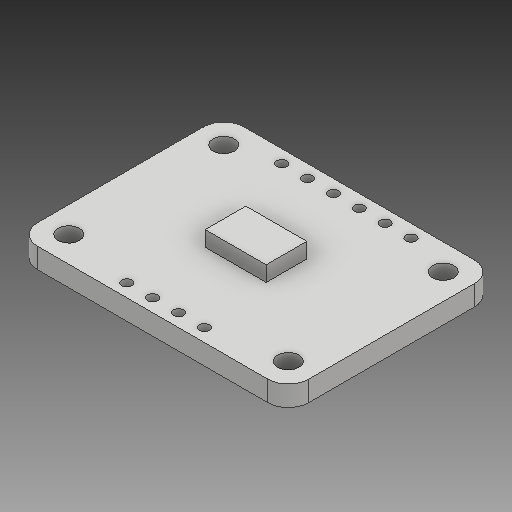
# Autodesk Inventor part: BNO055
Saved by Autodesk Inventor 2018 (Build 220112000, 112)
## iProperties
Part Number: BNO055
Material: Generisch
Document SubType Name: Modeling
Designer: Jochen Alt
Mass: 1.06958 g
Surface Area: 13.6029 cm^2
Volume: 1.06958 cm^3
Density: 1 g/cm^3
Appearance: Vorgabe
Author: Jochen Alt
Autodesk Inventor part; units mm, degrees
ref_plane "YZ Plane" through (0, 0, 0) normal (1, 0, 0) x (0, 1, 0)
ref_plane "XZ Plane" through (0, 0, 0) normal (0, 1, 0) x (-1, 0, 0)
ref_plane "XY Plane" through (0, 0, 0) normal (0, 0, 1) x (1, 0, 0)
sketch "Skizze1" plane through (0, 0, 0) normal (0, 0, 1) x (1, 0, 0)
  line L0 (-13.335, 10.16) -> (13.335, 10.16)
  line L1 (13.335, 10.16) -> (13.335, -10.16)
  line L2 (13.335, -10.16) -> (-13.335, -10.16)
  line L3 (-13.335, -10.16) -> (-13.335, 10.16)
  line L4 (-13.335, 10.16) -> (13.335, -10.16) construction
  line L5 (13.335, 10.16) -> (-13.335, -10.16) construction
  point P0 (0, 0)
  dimension "d0" = 26.67
  dimension "d1" = 20.32
  constraints: 12 end point, 2 midpoint, 2 parallel, 1 horizontal, 1 perpendicular
  measures "d0" distance of L1.end L2.end
  measures "d1" distance of L0.end L1.end
extrude "Extrusion1" add sketch "Skizze1" along normal blind 2
fillet "Rundung1" radius 2 4 edges at (-13.335, -10.16, 1) (13.335, -10.16, 1) (13.335, 10.16, 1) (-13.335, 10.16, 1)
sketch "Skizze2" plane through (0, 0, 0) normal (0, 0, -1) x (-1, 0, 0)
  line L0 (-10.795, -7.62) -> (10.795, -7.62) construction
  line L1 (10.795, -7.62) -> (10.795, 7.62) construction
  line L2 (10.795, 7.62) -> (-10.795, 7.62) construction
  line L3 (-10.795, 7.62) -> (-10.795, -7.62) construction
  line L4 (-10.795, -7.62) -> (10.795, 7.62) construction
  line L5 (10.795, -7.62) -> (-10.795, 7.62) construction
  line L6 (-6.35, -8.89) -> (6.35, -8.89) construction
  line L7 (6.35, -8.89) -> (6.35, 8.89) construction
  line L8 (6.35, 8.89) -> (-6.35, 8.89) construction
  line L9 (-6.35, 8.89) -> (-6.35, -8.89) construction
  line L10 (-6.35, -8.89) -> (6.35, 8.89) construction
  line L11 (6.35, -8.89) -> (-6.35, 8.89) construction
  circle A0 centre (6.35, 8.89) radius 0.5
  circle A1 centre (3.81, 8.89) radius 0.5
  line L12 (3.81, 8.89) -> (-8.89, 8.89) construction
  circle A2 centre (1.27, 8.89) radius 0.5
  line L13 (1.27, 8.89) -> (-11.43, 8.89) construction
  circle A3 centre (-1.27, 8.89) radius 0.5
  line L14 (-1.27, 8.89) -> (-13.97, 8.89) construction
  circle A4 centre (-3.81, 8.89) radius 0.5
  line L15 (-3.81, 8.89) -> (-16.51, 8.89) construction
  circle A5 centre (-6.35, 8.89) radius 0.5
  line L16 (-6.35, 8.89) -> (-19.05, 8.89) construction
  circle A6 centre (3.81, -8.89) radius 0.5
  circle A7 centre (1.27, -8.89) radius 0.5
  line L17 (-8.89, -8.89) -> (3.81, -8.89) construction
  circle A8 centre (-1.27, -8.89) radius 0.5
  line L18 (-11.43, -8.89) -> (1.27, -8.89) construction
  circle A9 centre (-3.81, -8.89) radius 0.5
  line L19 (-13.97, -8.89) -> (-1.27, -8.89) construction
  circle A10 centre (10.795, -7.62) radius 1.05
  circle A11 centre (-10.795, -7.62) radius 1.05
  circle A12 centre (-10.795, 7.62) radius 1.05
  circle A13 centre (10.795, 7.62) radius 1.05
  point P0 (0, 0)
  dimension "d5" = 21.59
  dimension "d6" = 15.24
  dimension "d7" = 17.78
  dimension "d8" = 12.7
  dimension "d9" = 1
  dimension "d14" = 2.54
  dimension "d19" = 1
  dimension "d22" = 2.54
  dimension "d27" = 2.1
  dimension "d28" = 2.1
  dimension "d29" = 2.1
  dimension "d30" = 2.1
  constraints: 40 end point, 14 centre point, 7 coincident, 4 horizontal, 4 midpoint, 4 parallel, 4 point on line, 2 collinear, 2 perpendicular, 38 other
  measures "d5" distance of L2.end L1.end
  measures "d6" distance between parallel lines of L2 L0
  measures "d7" distance of L7.end L6.end
  measures "d8" distance between parallel lines of L9 L7
  measures "d9" diameter of A0
  measures "d14" distance of A0.centre A1.centre
  measures "d19" diameter of A6
  measures "d22" distance of A6.centre A7.centre
  measures "d27" diameter of A10
  measures "d28" diameter of A11
  measures "d29" diameter of A12
  measures "d30" diameter of A13
extrude "Extrusion2" cut sketch "Skizze2" against normal through all
sketch "Skizze3" plane through (0, 0, 2) normal (0, 0, 1) x (1, 0, 0)
  line L0 (-3, 2) -> (3, 2)
  line L1 (3, 2) -> (3, -2)
  line L2 (3, -2) -> (-3, -2)
  line L3 (-3, -2) -> (-3, 2)
  line L4 (-3, 2) -> (3, -2) construction
  line L5 (3, 2) -> (-3, -2) construction
  point P0 (0, 0)
  dimension "d33" = 6
  dimension "d34" = 4
  constraints: 12 end point, 2 midpoint, 2 parallel, 1 horizontal, 1 perpendicular
  measures "d33" distance of L1.end L2.end
  measures "d34" distance of L0.end L1.end
extrude "Extrusion3" add sketch "Skizze3" along normal blind 1.5
